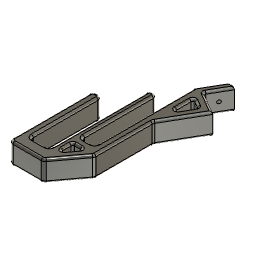
desk_side_laptop_hanger (Autodesk Fusion 360 design; units mm, degrees)
Autodesk Fusion 360 part; units mm, degrees
sketch "Sketch1" plane through (0, 0, 0) normal (0, 0, 1) x (1, 0, 0)
  line L0 (0, 0) -> (0, -100)
  line L1 (0, 0) -> (8, 0)
  line L2 (8, 0) -> (8, -90)
  line L3 (8, -90) -> (24, -90)
  line L4 (24, -90) -> (24, 30)
  line L5 (0, -100) -> (34, -100)
  line L6 (34, -100) -> (34, 30)
  line L7 (34, 30) -> (24, 30)
  line L8 (24, 30) -> (40, 57.712813)
  line L9 (40, 57.712813) -> (47.5, 53.382686)
  line L10 (47.5, 53.382686) -> (34, 30)
  line L11 (34, 30) -> (59.980762, 15)
  line L12 (59.980762, 15) -> (34, -30)
  line L13 (34, 18.452995) -> (46.320508, 11.339746)
  line L14 (46.320508, 11.339746) -> (34, -10)
  line L15 (8, -100) -> (8, -135)
  line L16 (8, -135) -> (-33, -135)
  line L17 (-33, -135) -> (-33, -35)
  line L18 (-33, -35) -> (-23, -35)
  line L19 (-23, -35) -> (-23, -120)
  line L20 (-23, -120) -> (0, -120)
  line L21 (0, -120) -> (0, -100)
  line L22 (34, -100) -> (8, -135)
  line L23 (21.542726, -100) -> (8, -118.230593)
  dimension "d1" = 100
  dimension "d2" = 8
  dimension "d3" = 16
  dimension "d4" = 10
  dimension "d5" = 10
  dimension "d6" = 120
  dimension "d7" = 30
  dimension "d8" = 27
  dimension "d9" = 30
  dimension "d10" = 10
  dimension "d11" = 10
  dimension "d12" = 8
  dimension "d13" = 15
  dimension "d14" = 10
  dimension "d15" = 23
  dimension "d16" = 10
  dimension "d18" = 120
  dimension "d19" = 100
  constraint coincident L0.start L1.start
  constraint vertical L0
  constraint perpendicular L0 L1
  constraint perpendicular L1 L2
  constraint perpendicular L2 L3
  constraint perpendicular L3 L4
  constraint perpendicular L0 L5
  constraint perpendicular L5 L6
  constraint perpendicular L4 L7
  constraint perpendicular L8 L9
  constraint parallel L8 L10
  constraint perpendicular L10 L11
  constraint coincident L6 L12.end
  constraint perpendicular L11 L12
  constraint coincident L6 L14.end
  constraint parallel L11 L13
  constraint parallel L12 L14
  constraint coincident L5 L15.start
  constraint perpendicular L5 L15
  constraint perpendicular L2 L16
  constraint perpendicular L16 L17
  constraint perpendicular L17 L18
  constraint perpendicular L18 L19
  constraint perpendicular L19 L20
  constraint collinear L0 L21
  constraint parallel L22 L23
  measures "d1" distance of L0.start L0.end
  measures "d2" distance of L0 L2
  measures "d3" distance of L2 L4
  measures "d4" distance of L3 L5
  measures "d5" distance of L4 L6
  measures "d6" distance of L3 L7
  measures "d7" angle of L4 L8
  measures "d8" distance of L6.end L9
  measures "d9" distance of L6.end L12
  measures "d10" distance of L11 L13
  measures "d11" distance of L12 L14
  measures "d12" distance of L15 L21
  measures "d13" distance of L16 L20
  measures "d14" distance of L17 L19
  measures "d15" distance of L19 L21
  measures "d16" distance of L22 L23
  measures "d18" distance of L1 L20
  measures "d19" distance of L16 L18
extrude "Extrude1" add sketch "Sketch1" along normal blind 25 contours L0 L1 L2 L3 L4 L5 L6 L7 | L5 L15 L16 L17 L18 L19 L20 L21 | L5 L15 L22 L23 | L7 L8 L9 L10 | L6 L11 L12 L13 L14 picked at (27.333333, -30) picked at (-16, -130) picked at (16.666667, -117.743531) picked at (32.666667, 39.237604) picked at (42.660254, -8.333333)
fillet "Fillet1" radius 5 1 edges at (40, 57.712813, 12.5)
fillet "Fillet2" radius 2 3 edges at (34, 18.452995, 12.5) (34, -10, 12.5) (46.320508, 11.339746, 12.5)
fillet "Fillet3" radius 2 1 edges at (34, 30, 12.5)
fillet "Fillet4" radius 5 1 edges at (24, 30, 12.5)
fillet "Fillet5" radius 2 3 edges at (8, -100, 12.5) (21.542726, -100, 12.5) (8, -118.230593, 12.5)
fillet "Fillet6" radius 4 8 edges at (8, 0, 12.5) (0, 0, 12.5) (-23, -35, 12.5) (-33, -35, 12.5) (24, -90, 12.5) (8, -90, 12.5) (0, -120, 12.5) (-23, -120, 12.5)
fillet "Fillet7" radius 5 4 edges at (-33, -135, 12.5) (8, -135, 12.5) (34, -100, 12.5) (34, -30, 12.5)
sketch "Sketch3" plane through (12.509619, -7.222432, 0) normal (0.866025, -0.5, 0) x (0.5, 0.866025, 0)
  line L0 (44.980762, 25) -> (44.980762, 0)
  line L1 (44.980762, 0) -> (69.980762, 0)
  line L2 (69.980762, 0) -> (69.980762, 25)
  line L3 (69.980762, 25) -> (44.980762, 25)
  circle A0 centre (56.480762, 12.5) radius 2
  dimension "d38" = 4
  dimension "d39" = 12.5
  dimension "d40" = 13.5
  measures "d38" diameter of A0
extrude "Extrude2" cut sketch "Sketch3" against normal blind 23 contours A0 picked at (56.233888, 13.164803)
ref_plane "WorkPlane1" through (13.490381, -38.643594, 12.5) normal (0, 0, -1) x (-1, 0, 0)
sketch "Sketch4" plane through (13.490381, -38.643594, 12.5) normal (0, 0, -1) x (-1, 0, 0)
  line L0 (-20.759619, 86.397114) -> (-18.759619, 82.933013)
  line L1 (-20.759619, 86.397114) -> (-22.009619, 88.562178)
  line L2 (-22.009619, 88.562178) -> (-23.107695, 84.464102)
  line L3 (-23.107695, 84.464102) -> (-22.357695, 83.165064)
  line L4 (-22.357695, 83.165064) -> (-19.759619, 84.665064)
  dimension "d43" = 3
  dimension "d44" = 4.5
  dimension "d45" = 45
  constraint parallel L0 L1
  constraint parallel L0 L3
  constraint perpendicular L0 L4
  measures "d43" distance of L0 L3
  measures "d45" angle of L1 L2
revolve "Revolve1" cut sketch "Sketch4" angle 360 about axis through (35.848076, 44.52147, 12.5) along (-0.866025, 0.5, 0)
sketch "Sketch5" plane through (24, 0, 0) normal (-1, 0, 0) x (0, -1, 0)
  line L0 (86, 25) -> (-28.660254, 25)
  line L1 (-28.660254, 25) -> (-28.660254, 0)
  line L2 (-28.660254, 0) -> (86, 0)
  circle A0 centre (-21.660254, 12.5) radius 2
  line L3 (86, 0) -> (86, 25)
  dimension "d47" = 4
  dimension "d48" = 12.5
  dimension "d49" = 7
  measures "d47" diameter of A0
extrude "Extrude3" cut sketch "Sketch5" against normal blind 44 contours A0 picked at (-22.275131, 12.400638)
sketch "Sketch6" plane through (13.490381, -38.643594, 12.5) normal (0, 0, -1) x (-1, 0, 0)
  line L0 (-10.509619, 62.303848) -> (-10.509619, 58.303848)
  line L1 (-10.509619, 62.303848) -> (-10.509619, 64.803848)
  line L2 (-10.509619, 64.803848) -> (-13.509619, 61.803848)
  line L3 (-13.509619, 61.803848) -> (-13.509619, 60.303848)
  line L4 (-13.509619, 60.303848) -> (-10.509619, 60.303848)
  dimension "d52" = 4.5
  dimension "d53" = 3
  dimension "d54" = 45
  constraint parallel L0 L1
  constraint parallel L0 L3
  constraint perpendicular L0 L4
  measures "d54" angle of L1 L2
revolve "Revolve2" cut sketch "Sketch6" angle 360 about axis through (27, 21.660254, 12.5) along (-1, 0, 0)
fillet "Fillet8" radius 2.5 2 faces at (-8.83785, -130, 25) (-8.83785, -130, 0)
named bodies: "desk_side_laptop_hanger"
